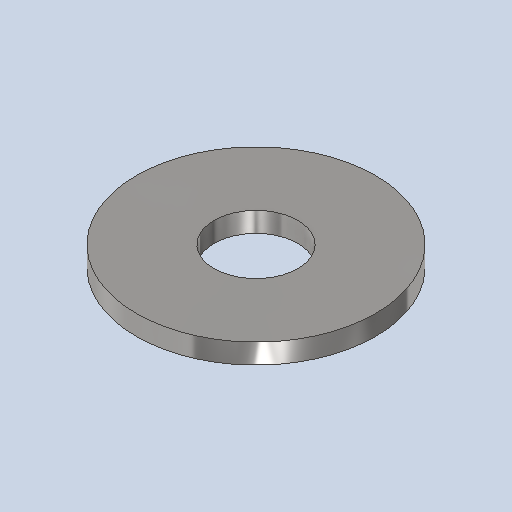
# Autodesk Inventor part: UUW-0412-10H
Saved by Autodesk Inventor 2024.2 (Build 282272000, 272)
## iProperties
Created: 2024-01-03
Part Number: UUW-0412-10H
Material: Stainless Steel AISI 304
Document SubType Name: Modeling
Designer: Masato Kubotera
Density: 8 g/cm^3
Appearance: Steel - Polished
Catalog Web Link: https://www.hirosugi-net.co.jp/shop/g/g58926/
Vendor: HIROSUGI
Author: Masato Kubotera
Autodesk Inventor part; units mm, degrees
ref_plane "YZ Plane" through (0, 0, 0) normal (1, 0, 0) x (0, 1, 0)
ref_plane "XZ Plane" through (0, 0, 0) normal (0, 1, 0) x (-1, 0, 0)
ref_plane "XY Plane" through (0, 0, 0) normal (0, 0, 1) x (1, 0, 0)
sketch "Sketch1" plane through (0, 0, 0) normal (0, 1, 0) x (-1, 0, 0)
  line L0 (0, 0) -> (0, 1)
  line L1 (-2.1, 1) -> (-2.1, 0)
  line L2 (-2.1, 0) -> (-6, 0)
  line L3 (-6, 0) -> (-6, 1)
  line L4 (-6, 1) -> (-2.1, 1)
  dimension "InsideDiameter" = 4.2
  dimension "OuterDiameter" = 12
  dimension "Thickness" = 1
  constraints: 10 end point, 3 vertical, 2 horizontal, 2 point on line
  measures "InsideDiameter" diameter of L1 L0
  measures "OuterDiameter" diameter of L3 L0
  measures "Thickness" distance of L2.end L3.end
revolve "Revolution1" add sketch "Sketch1" angle 360 about axis through (0, 0, 0) along (0, 0, 1)
body "Solid1"
